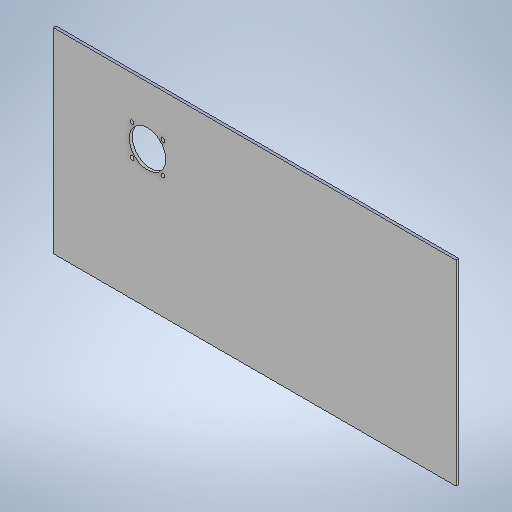
# Autodesk Inventor part: BackWall
Saved by Autodesk Inventor 2026.2 (Build 302298010, 298A)
## iProperties
Created: 2026-03-19
Part Number: BackWall
Material: Ogólny
Document SubType Name: Modeling
Designer: Patryk
Density: 1 g/cm^3
Appearance: Domyślna
Author: Patryk
Autodesk Inventor part; units mm, degrees
ref_plane "YZ Plane" through (0, 0, 0) normal (1, 0, 0) x (0, 1, 0)
ref_plane "XZ Plane" through (0, 0, 0) normal (0, 1, 0) x (-1, 0, 0)
ref_plane "XY Plane" through (0, 0, 0) normal (0, 0, 1) x (1, 0, 0)
sketch "Szkic1" plane through (0, 0, 0) normal (0, 0, 1) x (1, 0, 0)
  line L0 (209, 101.5) -> (-209, 101.5)
  line L1 (-209, 101.5) -> (-209, -101.5)
  line L2 (-209, -101.5) -> (209, -101.5)
  line L3 (209, -101.5) -> (209, 101.5)
  line L4 (209, 101.5) -> (-209, -101.5) construction
  line L5 (-209, 101.5) -> (209, -101.5) construction
  point P0 (0, 0)
  dimension "d0" = 418
  dimension "d1" = 203
  constraints: 12 end point, 2 midpoint, 2 parallel, 1 horizontal, 1 perpendicular
  measures "d0" distance of L2.end L1.end
  measures "d1" distance of L1.end L0.end
extrude "Wyciągnięcie proste1" add sketch "Szkic1" along normal mid plane 3
sketch "Szkic2" plane through (0, 0, 1.5) normal (0, 0, 1) x (1, 0, 0)
  circle A0 centre (-111, 41.5) radius 19
  line L0 (-209, 101.5) -> (-209, -101.5) projected
  line L1 (209, 101.5) -> (-209, 101.5) projected
  line L2 (-95, 25.5) -> (-127, 25.5)
  line L3 (-127, 25.5) -> (-127, 57.5)
  line L4 (-127, 57.5) -> (-95, 57.5)
  line L5 (-95, 57.5) -> (-95, 25.5)
  circle A1 centre (-127, 57.5) radius 2
  circle A2 centre (-95, 57.5) radius 2
  circle A3 centre (-95, 25.5) radius 2
  circle A4 centre (-127, 25.5) radius 2
  line L6 (-209, -101.5) -> (209, -101.5) projected
  line L7 (209, -101.5) -> (209, 101.5) projected
  line L8 (-209, 80.5) -> (-209, 91.5)
  point P0 (0, 0)
  dimension "d7" = 32
  dimension "d8" = 32
  dimension "d9" = 4
  dimension "d10" = 4
  dimension "d12" = 4
  dimension "d105" = 38
  dimension "d106" = 44
  dimension "d107" = 304
  dimension "d108" = 60
  dimension "d109" = 320
  dimension "d110" = 10
  dimension "d111" = 21
  constraints: 10 end point, 5 centre point, 4 coincident, 3 parallel, 1 equal radius, 1 horizontal, 1 perpendicular, 1 point on line
  measures "d7" distance of L3.end L4.end
  measures "d8" distance of L2.end L3.end
  measures "d9" diameter of A1
  measures "d10" diameter of A2
  measures "d12" diameter of A4
  measures "d105" diameter of A0
  measures "d106" distance between parallel lines of L1 L4
  measures "d107" distance between parallel lines of L7 L5
  measures "d108" distance from line of A0.centre L1
  measures "d109" distance from line of A0.centre L7
  measures "d110" distance from line of L8.end L1
  measures "d111" distance from line of L8.start L1
extrude "Wyciągnięcie proste3" cut sketch "Szkic2" against normal through all contours A2 L4 L5 | L5 L4 A2 | A3 L2 L5 | L5 L2 A3 | A1 L3 L4 | L4 L3 A1 | A4 L3 L2 | L2 L3 A4
extrude "Wyciągnięcie proste4" cut sketch "Szkic2" against normal through all contours A0 L5 | L5 A0 L2 L3 L4 | L4 A0 | A0 L2 | L3 A0
